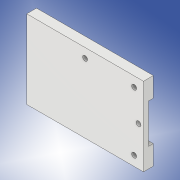
# Autodesk Inventor part: SP004
Saved by Autodesk Inventor 2017 SP1 (Build 210196100, 196)
## iProperties
Created: 2017-08-09
Part Number: SP004
Material: ABS Plastic
Document SubType Name: Modeling
Designer: Zach
Density: 1.06 g/cm^3
Appearance: CR White
Author: Zach
Autodesk Inventor part; units mm, degrees
ref_plane "YZ Plane" through (0, 0, 0) normal (1, 0, 0) x (0, 1, 0)
ref_plane "XZ Plane" through (0, 0, 0) normal (0, 1, 0) x (-1, 0, 0)
ref_plane "XY Plane" through (0, 0, 0) normal (0, 0, 1) x (1, 0, 0)
sketch "Sketch1" plane through (0, 0, 0) normal (0, 0, 1) x (1, 0, 0)
  line L0 (0, 0) -> (119, 0)
  line L1 (119, 0) -> (119, 80)
  line L2 (119, 80) -> (0, 80)
  line L3 (0, 80) -> (0, 0)
  dimension "d0" = 119
  dimension "d1" = 80
  constraints: 8 end point, 2 parallel, 1 horizontal, 1 perpendicular
  measures "d0" distance of L2.end L1.end
  measures "d1" distance of L1.end L0.end
extrude "Extrusion1" add sketch "Sketch1" along normal blind 10
sketch "Sketch2" plane through (0, 0, 10) normal (0, 0, 1) x (1, 0, 0)
  circle A0 centre (109.5, 70) radius 2.5
  circle A1 centre (109.5, 10) radius 2.5
  line L0 (119, 80) -> (0, 80) projected
  line L1 (119, 0) -> (119, 80) projected
  point P0 (0, 0)
  dimension "d4" = 5
  dimension "d5" = 5
  dimension "d6" = 10
  dimension "d7" = 60
  dimension "d8" = 9.5
  constraints: 2 centre point, 1 vertical alignment
  measures "d4" diameter of A0
  measures "d5" diameter of A1
  measures "d6" distance from line of L0 A0.centre
  measures "d7" distance of A0.centre A1.centre
  measures "d8" distance from line of L1 A0.centre
extrude "Extrusion2" cut sketch "Sketch2" against normal through all
sketch "Sketch3" plane through (0, 0, 0) normal (0, 0, -1) x (-1, 0, 0)
  line L0 (-119, 0) -> (-119, 80) projected
  line L1 (-119, 60) -> (-109, 60)
  line L2 (-109, 60) -> (-109, 20)
  line L3 (-109, 20) -> (-119, 20)
  line L4 (-119, 20) -> (-119, 60)
  line L5 (-119, 80) -> (0, 80) projected
  point P0 (0, 0)
  dimension "d11" = 10
  dimension "d12" = 40
  dimension "d13" = 20
  constraints: 8 end point, 2 parallel, 1 horizontal, 1 perpendicular, 1 point on line
  measures "d11" distance of L2.end L3.end
  measures "d12" distance of L1.end L2.end
  measures "d13" distance between parallel lines of L1 L5
extrude "Extrusion3" cut sketch "Sketch3" against normal blind 5
sketch "Sketch4" plane through (0, 0, 5) normal (0, 0, -1) x (-1, 0, 0)
  line L0 (-109, 60) -> (-119, 60)
  line L1 (-119, 60) -> (-119, 20)
  line L2 (-119, 20) -> (-109, 20)
  line L3 (-109, 20) -> (-109, 60)
  line L4 (-119, 80) -> (0, 80) projected
  line L5 (-119, 0) -> (-119, 80) projected
  circle A0 centre (-114, 40) radius 2.5
  point P0 (0, 0)
  point P1 (-119, 20)
  point P2 (-119, 40)
  point P3 (-114, 60)
  point P4 (-119, 40)
  dimension "d18" = 10
  dimension "d19" = 40
  dimension "d20" = 20
  dimension "d21" = 5
  constraints: 8 end point, 4 midpoint, 2 parallel, 1 centre point, 1 horizontal, 1 horizontal alignment, 1 perpendicular, 1 vertical alignment
  measures "d18" distance of L2.end L1.end
  measures "d19" distance of L1.end L0.end
  measures "d20" distance between parallel lines of L4 L0
  measures "d21" diameter of A0
extrude "Extrusion4" cut sketch "Sketch4" against normal through all contours A0
sketch "Sketch5" plane through (0, 0, 10) normal (0, 0, 1) x (1, 0, 0)
  circle A0 centre (59.5, 70.5) radius 2.5
  line L0 (119, 80) -> (0, 80) projected
  point P0 (0, 0)
  point P1 (59.5, 80)
  dimension "d24" = 5
  dimension "d25" = 9.5
  constraints: 1 centre point, 1 midpoint, 1 vertical alignment
  measures "d24" diameter of A0
  measures "d25" distance from line of L0 A0.centre
extrude "Extrusion5" cut sketch "Sketch5" against normal through all
body "Solid1"
